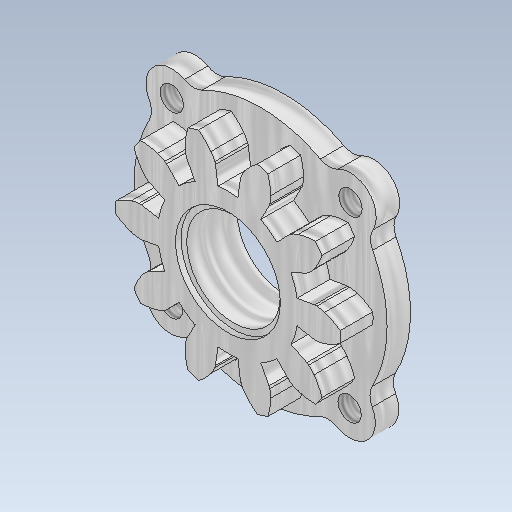
# Autodesk Inventor part: ｍ2歯数10ギア甲d10
Saved by Autodesk Inventor 2020.2 (Build 242310000, 310)
## iProperties
Created: 2019-11-09
Part Number: ｍ2歯数10ギア甲d10
Material: アルミニウム 7075
Document SubType Name: Modeling
Designer: aoyam
Density: 2.81 g/cm^3
Appearance: サテン - ブラシ仕上げ 重厚
Author: aoyam
Autodesk Inventor part; units mm, degrees
ref_plane "YZ Plane" through (0, 0, 0) normal (1, 0, 0) x (0, 1, 0)
ref_plane "XZ Plane" through (0, 0, 0) normal (0, 1, 0) x (-1, 0, 0)
ref_plane "XY Plane" through (0, 0, 0) normal (0, 0, 1) x (1, 0, 0)
sketch "スケッチ1" plane through (0, 0, 0) normal (0, 0, 1) x (1, 0, 0)
  arc A0 (-6.7711, 4.8044) -> (-6.8414, 4.5719) centre (-5.6655, 4.3429) ccw
  arc A1 (-6.3619, 5.5344) -> (-6.7711, 4.8044) centre (-3.6713, 3.5464) ccw
  arc A2 (-5.0279, 6.8503) -> (-6.3619, 5.5344) centre (-1.5449, 1.9856) ccw
  arc A3 (-9.5045, 4.5719) -> (-9.5748, 4.8044) centre (-10.6804, 4.3429) ccw
  arc A4 (-9.5748, 4.8044) -> (-9.984, 5.5344) centre (-12.6746, 3.5464) ccw
  arc A5 (-9.984, 5.5344) -> (-11.318, 6.8503) centre (-14.801, 1.9856) ccw
  arc A6 (-7.1102, 2.6941) -> (-9.2357, 2.6941) centre (-8.1729, -4.7302) ccw
  arc A7 (-11.318, 6.8503) -> (-12.4354, 6.4873) centre (-8.1729, -4.7302) ccw
  line L0 (-7.1102, 2.6941) -> (-6.8414, 4.5719)
  line L1 (-9.2357, 2.6941) -> (-9.5045, 4.5719)
  line L2 (-22.1729, -4.7302) -> (5.8271, -4.7302)
  line L3 (-8.1729, -18.7302) -> (-8.1729, 9.2698)
  arc A8 (-11.6771, 1.9009) -> (-13.3966, 0.6516) centre (-8.1729, -4.7302) ccw
  line L4 (-11.6771, 1.9009) -> (-12.5634, 3.578)
  line L5 (-13.3966, 0.6516) -> (-14.7178, 2.0127)
  arc A9 (-14.7178, 2.0127) -> (-14.9114, 2.1595) centre (-15.5346, 1.1363) ccw
  arc A10 (-12.4354, 6.4873) -> (-12.7411, 4.6385) centre (-6.7582, 4.5989) ccw
  arc A11 (-14.9114, 2.1595) -> (-15.6715, 2.5095) centre (-16.6797, -0.6803) ccw
  arc A12 (-15.6715, 2.5095) -> (-17.5242, 2.7901) centre (-17.4826, -3.1929) ccw
  arc A13 (-17.5242, 2.7901) -> (-18.2148, 1.8395) centre (-8.1729, -4.7302) ccw
  arc A14 (-12.6431, 3.8075) -> (-12.5634, 3.578) centre (-11.4774, 4.084) ccw
  arc A15 (-12.7411, 4.6385) -> (-12.6431, 3.8075) centre (-9.3959, 4.6117) ccw
  arc A16 (-14.9055, -1.4252) -> (-15.5623, -3.4467) centre (-8.1729, -4.7302) ccw
  line L6 (-14.9055, -1.4252) -> (-16.6083, -0.5893)
  line L7 (-15.5623, -3.4467) -> (-17.4312, -3.122)
  arc A17 (-17.4312, -3.122) -> (-17.6741, -3.1171) centre (-17.5768, -4.3112) ccw
  arc A18 (-18.2148, 1.8395) -> (-17.3755, 0.1642) centre (-12.5119, 3.6488) ccw
  arc A19 (-17.6741, -3.1171) -> (-18.4948, -3.2807) centre (-17.4355, -6.4539) ccw
  arc A20 (-18.4948, -3.2807) -> (-20.1586, -4.1427) centre (-16.6083, -8.9586) ccw
  arc A21 (-20.1586, -4.1427) -> (-20.1586, -5.3177) centre (-8.1729, -4.7302) ccw
  arc A22 (-16.8077, -0.4506) -> (-16.6083, -0.5893) centre (-16.0272, 0.4583) ccw
  arc A23 (-17.3755, 0.1642) -> (-16.8077, -0.4506) centre (-14.6534, 2.1087) ccw
  arc A24 (-15.5623, -6.0137) -> (-14.9055, -8.0351) centre (-8.1729, -4.7302) ccw
  line L8 (-15.5623, -6.0137) -> (-17.4312, -6.3384)
  line L9 (-14.9055, -8.0351) -> (-16.6083, -8.871)
  arc A25 (-16.6083, -8.871) -> (-16.8077, -9.0098) centre (-16.0272, -9.9187) ccw
  arc A26 (-20.1586, -5.3177) -> (-18.4948, -6.1797) centre (-16.6083, -0.5018) ccw
  arc A27 (-16.8077, -9.0098) -> (-17.3755, -9.6246) centre (-14.6534, -11.5691) ccw
  arc A28 (-17.3755, -9.6246) -> (-18.2148, -11.2999) centre (-12.5119, -13.1092) ccw
  arc A29 (-18.2148, -11.2999) -> (-17.5242, -12.2504) centre (-8.1729, -4.7302) ccw
  arc A30 (-17.6741, -6.3433) -> (-17.4312, -6.3384) centre (-17.5768, -5.1492) ccw
  arc A31 (-18.4948, -6.1797) -> (-17.6741, -6.3433) centre (-17.4355, -3.0065) ccw
  arc A32 (-13.3966, -10.1119) -> (-11.6771, -11.3612) centre (-8.1729, -4.7302) ccw
  line L10 (-13.3966, -10.1119) -> (-14.7178, -11.4731)
  line L11 (-11.6771, -11.3612) -> (-12.5634, -13.0384)
  arc A33 (-12.5634, -13.0384) -> (-12.6431, -13.2679) centre (-11.4774, -13.5443) ccw
  arc A34 (-17.5242, -12.2504) -> (-15.6715, -11.9699) centre (-17.4826, -6.2675) ccw
  arc A35 (-12.6431, -13.2679) -> (-12.7411, -14.0989) centre (-9.3959, -14.0721) ccw
  arc A36 (-12.7411, -14.0989) -> (-12.4354, -15.9476) centre (-6.7582, -14.0593) ccw
  arc A37 (-12.4354, -15.9476) -> (-11.318, -16.3107) centre (-8.1729, -4.7302) ccw
  arc A38 (-14.9114, -11.6198) -> (-14.7178, -11.4731) centre (-15.5346, -10.5967) ccw
  arc A39 (-15.6715, -11.9699) -> (-14.9114, -11.6198) centre (-16.6797, -8.7801) ccw
  arc A40 (-9.2357, -12.1545) -> (-7.1102, -12.1545) centre (-8.1729, -4.7302) ccw
  line L12 (-9.2357, -12.1545) -> (-9.5045, -14.0323)
  line L13 (-7.1102, -12.1545) -> (-6.8414, -14.0323)
  arc A41 (-6.8414, -14.0323) -> (-6.7711, -14.2648) centre (-5.6655, -13.8033) ccw
  arc A42 (-11.318, -16.3107) -> (-9.984, -14.9948) centre (-14.801, -11.446) ccw
  arc A43 (-6.7711, -14.2648) -> (-6.3619, -14.9948) centre (-3.6713, -13.0068) ccw
  arc A44 (-6.3619, -14.9948) -> (-5.0279, -16.3107) centre (-1.5449, -11.446) ccw
  arc A45 (-5.0279, -16.3107) -> (-3.9105, -15.9476) centre (-8.1729, -4.7302) ccw
  arc A46 (-9.5748, -14.2648) -> (-9.5045, -14.0323) centre (-10.6804, -13.8033) ccw
  arc A47 (-9.984, -14.9948) -> (-9.5748, -14.2648) centre (-12.6746, -13.0068) ccw
  arc A48 (-4.6688, -11.3612) -> (-2.9493, -10.1119) centre (-8.1729, -4.7302) ccw
  line L14 (-4.6688, -11.3612) -> (-3.7825, -13.0384)
  line L15 (-2.9493, -10.1119) -> (-1.6281, -11.4731)
  arc A49 (-1.6281, -11.4731) -> (-1.4345, -11.6198) centre (-0.8113, -10.5967) ccw
  arc A50 (-3.9105, -15.9476) -> (-3.6048, -14.0989) centre (-9.5877, -14.0593) ccw
  arc A51 (-1.4345, -11.6198) -> (-0.6744, -11.9699) centre (0.3338, -8.7801) ccw
  arc A52 (-0.6744, -11.9699) -> (1.1783, -12.2504) centre (1.1367, -6.2675) ccw
  arc A53 (1.1783, -12.2504) -> (1.8689, -11.2999) centre (-8.1729, -4.7302) ccw
  arc A54 (-3.7028, -13.2679) -> (-3.7825, -13.0384) centre (-4.8685, -13.5443) ccw
  arc A55 (-3.6048, -14.0989) -> (-3.7028, -13.2679) centre (-6.95, -14.0721) ccw
  arc A56 (-1.4404, -8.0351) -> (-0.7836, -6.0137) centre (-8.1729, -4.7302) ccw
  line L16 (-1.4404, -8.0351) -> (0.2624, -8.871)
  line L17 (-0.7836, -6.0137) -> (1.0853, -6.3384)
  arc A57 (1.0853, -6.3384) -> (1.3282, -6.3433) centre (1.2309, -5.1492) ccw
  arc A58 (1.8689, -11.2999) -> (1.0296, -9.6246) centre (-3.834, -13.1092) ccw
  arc A59 (1.3282, -6.3433) -> (2.1489, -6.1797) centre (1.0897, -3.0065) ccw
  arc A60 (2.1489, -6.1797) -> (3.8127, -5.3177) centre (0.2624, -0.5018) ccw
  arc A61 (3.8127, -5.3177) -> (3.8127, -4.1427) centre (-8.1729, -4.7302) ccw
  arc A62 (0.4618, -9.0098) -> (0.2624, -8.871) centre (-0.3187, -9.9187) ccw
  arc A63 (1.0296, -9.6246) -> (0.4618, -9.0098) centre (-1.6925, -11.5691) ccw
  arc A64 (-0.7836, -3.4467) -> (-1.4404, -1.4252) centre (-8.1729, -4.7302) ccw
  line L18 (-0.7836, -3.4467) -> (1.0853, -3.122)
  line L19 (-1.4404, -1.4252) -> (0.2624, -0.5893)
  arc A65 (0.2624, -0.5893) -> (0.4618, -0.4506) centre (-0.3187, 0.4583) ccw
  arc A66 (3.8127, -4.1427) -> (2.1489, -3.2807) centre (0.2624, -8.9586) ccw
  arc A67 (0.4618, -0.4506) -> (1.0296, 0.1642) centre (-1.6925, 2.1087) ccw
  arc A68 (1.0296, 0.1642) -> (1.8689, 1.8395) centre (-3.834, 3.6488) ccw
  arc A69 (1.8689, 1.8395) -> (1.1783, 2.7901) centre (-8.1729, -4.7302) ccw
  arc A70 (1.3282, -3.1171) -> (1.0853, -3.122) centre (1.2309, -4.3112) ccw
  arc A71 (2.1489, -3.2807) -> (1.3282, -3.1171) centre (1.0897, -6.4539) ccw
  arc A72 (-2.9493, 0.6516) -> (-4.6688, 1.9009) centre (-8.1729, -4.7302) ccw
  line L20 (-2.9493, 0.6516) -> (-1.6281, 2.0127)
  line L21 (-4.6688, 1.9009) -> (-3.7825, 3.578)
  arc A73 (-3.7825, 3.578) -> (-3.7028, 3.8075) centre (-4.8685, 4.084) ccw
  arc A74 (1.1783, 2.7901) -> (-0.6744, 2.5095) centre (1.1367, -3.1929) ccw
  arc A75 (-3.7028, 3.8075) -> (-3.6048, 4.6385) centre (-6.95, 4.6117) ccw
  arc A76 (-3.6048, 4.6385) -> (-3.9105, 6.4873) centre (-9.5877, 4.5989) ccw
  arc A77 (-3.9105, 6.4873) -> (-5.0279, 6.8503) centre (-8.1729, -4.7302) ccw
  arc A78 (-1.4345, 2.1595) -> (-1.6281, 2.0127) centre (-0.8113, 1.1363) ccw
  arc A79 (-0.6744, 2.5095) -> (-1.4345, 2.1595) centre (0.3338, -0.6803) ccw
  circle A80 centre (-8.1729, -4.7302) radius 2.5
  circle A81 centre (-8.1729, -4.7302) radius 5
  line L22 (-8.1729, -4.7302) -> (-17.6741, 4.8603) construction
  circle A82 centre (-17.6741, 4.8603) radius 1.25
  arc A83 (-16.7463, 5.698) -> (-18.5204, 3.9404) centre (-8.1729, -4.7302) ccw
  arc A84 (-20.0773, 1.6367) -> (-14.4281, 7.2332) centre (-8.1729, -4.7302) ccw
  arc A85 (-16.3313, 7.2602) -> (-20.0865, 3.5401) centre (-17.6741, 4.8603) ccw
  arc A86 (-16.3313, 7.2602) -> (-14.4281, 7.2332) centre (-15.3548, 9.0056) ccw
  arc A87 (-20.0773, 1.6367) -> (-20.0865, 3.5401) centre (-21.8409, 2.5799) ccw
  arc A88 (-20.1633, -12.8886) -> (-20.1364, -10.9853) centre (-21.9087, -11.912) ccw
  arc A89 (-20.1633, -12.8886) -> (-16.4432, -16.6437) centre (-17.7635, -14.2313) ccw
  circle A90 centre (-17.7635, -14.2313) radius 1.25
  arc A91 (-14.5398, -16.6345) -> (-16.4432, -16.6437) centre (-15.483, -18.3981) ccw
  arc A92 (-0.0146, -16.7206) -> (-1.9178, -16.6936) centre (-0.9911, -18.466) ccw
  arc A93 (-0.0146, -16.7206) -> (3.7406, -13.0004) centre (1.3282, -14.3207) ccw
  circle A94 centre (1.3282, -14.3207) radius 1.25
  arc A95 (3.7314, -11.097) -> (3.7406, -13.0004) centre (5.495, -12.0403) ccw
  arc A96 (3.8175, 3.4282) -> (3.7905, 1.5249) centre (5.5628, 2.4516) ccw
  arc A97 (3.8175, 3.4282) -> (0.0973, 7.1833) centre (1.4176, 4.771) ccw
  circle A98 centre (1.4176, 4.771) radius 1.25
  arc A99 (-1.8061, 7.1742) -> (0.0973, 7.1833) centre (-0.8629, 8.9378) ccw
  circle A100 centre (-8.1729, -4.7302) radius 5.6
  point P0 (0, 0)
  point P1 (-16.4019, 6.5961)
  point P2 (-21.4877, -0.4039)
  point P3 (-21.4877, -9.0564)
  point P4 (-16.4019, -16.0564)
  point P5 (-8.1729, -18.7302)
  point P6 (0.056, -16.0564)
  point P7 (5.1418, -9.0564)
  point P8 (5.1418, -0.4039)
  point P9 (0.056, 6.5961)
  point P10 (-18.4948, -3.2807)
  point P11 (-20.1586, -4.1427)
  point P12 (-20.1586, -5.3177)
  point P13 (-18.4948, -6.1797)
  point P14 (-17.6741, -6.3433)
  point P15 (-17.4312, -6.3384)
  point P16 (-15.5623, -6.0137)
  point P17 (-14.9055, -8.0351)
  point P18 (-16.8077, -9.0098)
  point P19 (-17.3755, -9.6246)
  point P20 (-18.2148, -11.2999)
  point P21 (-17.5242, -12.2504)
  point P22 (-15.6715, -11.9699)
  point P23 (-14.9114, -11.6198)
  point P24 (-13.3966, -10.1119)
  point P25 (-11.6771, -11.3612)
  point P26 (-12.5634, -13.0384)
  point P27 (-12.6431, -13.2679)
  point P28 (-12.7411, -14.0989)
  point P29 (-12.4354, -15.9476)
  point P30 (-11.318, -16.3107)
  point P31 (-9.984, -14.9948)
  point P32 (-9.5748, -14.2648)
  point P33 (-9.5045, -14.0323)
  point P34 (-9.2357, -12.1545)
  point P35 (-7.1102, -12.1545)
  point P36 (-6.7711, -14.2648)
  point P37 (-6.3619, -14.9948)
  point P38 (-5.0279, -16.3107)
  point P39 (-3.9105, -15.9476)
  point P40 (-3.6048, -14.0989)
  point P41 (-3.7028, -13.2679)
  point P42 (-3.7825, -13.0384)
  point P43 (-4.6688, -11.3612)
  point P44 (-2.9493, -10.1119)
  point P45 (-1.4345, -11.6198)
  point P46 (-0.6744, -11.9699)
  point P47 (1.1783, -12.2504)
  point P48 (1.8689, -11.2999)
  point P49 (1.0296, -9.6246)
  point P50 (0.4618, -9.0098)
  point P51 (0.2624, -8.871)
  point P52 (-1.4404, -8.0351)
  point P53 (-0.7836, -6.0137)
  point P54 (1.0853, -6.3384)
  point P55 (1.3282, -6.3433)
  point P56 (2.1489, -6.1797)
  point P57 (3.8127, -5.3177)
  point P58 (3.8127, -4.1427)
  point P59 (2.1489, -3.2807)
  point P60 (1.3282, -3.1171)
  point P61 (1.0853, -3.122)
  point P62 (-0.7836, -3.4467)
  point P63 (0.4618, -0.4506)
  point P64 (1.0296, 0.1642)
  point P65 (1.8689, 1.8395)
  point P66 (1.1783, 2.7901)
  point P67 (-0.6744, 2.5095)
  point P68 (-1.4345, 2.1595)
  point P69 (-1.6281, 2.0127)
  point P70 (-2.9493, 0.6516)
  point P71 (-4.6688, 1.9009)
  point P72 (-3.7825, 3.578)
  point P73 (-3.7028, 3.8075)
  point P74 (-3.6048, 4.6385)
  point P75 (-3.9105, 6.4873)
  point P76 (-5.0279, 6.8503)
  point P77 (-6.3619, 5.5344)
  point P78 (-6.7711, 4.8044)
  point P79 (-6.8414, 4.5719)
  point P80 (-7.1102, 2.6941)
  point P81 (-9.2357, 2.6941)
  point P82 (-9.5045, 4.5719)
  point P83 (-9.5748, 4.8044)
  point P84 (-9.984, 5.5344)
  point P85 (-11.318, 6.8503)
  point P86 (-12.4354, 6.4873)
  point P87 (-12.7411, 4.6385)
  point P88 (-12.6431, 3.8075)
  point P89 (-14.9114, 2.1595)
  point P90 (-15.6715, 2.5095)
  point P91 (-17.5242, 2.7901)
  point P92 (-18.2148, 1.8395)
  point P93 (-17.3755, 0.1642)
  point P94 (-16.8077, -0.4506)
  point P95 (-17.6741, -3.1171)
  point P96 (-18.6011, -13.3036)
  point P97 (-16.8436, -15.0777)
  point P98 (0.4004, -15.1584)
  point P99 (2.1745, -13.4008)
  point P100 (2.2552, 3.8432)
  point P101 (0.4977, 5.6173)
  point P102 (-1.9178, -16.6936)
  point P103 (3.7905, 1.5249)
  point P104 (-1.8061, 7.1742)
  point P105 (-20.1364, -10.9853)
  dimension "d2" = 360
  dimension "d6" = 5
  dimension "d8" = 10
  dimension "d9" = 13.5
  dimension "d10" = 2.5
  dimension "d13" = 2
  dimension "d16" = 360
  dimension "d20" = 0.6
  constraints: 196 point on circle, 101 centre point, 46 end point, 5 coincident, 4 tangent, 1 equal radius, 1 midpoint, 442 other
  measures "d6" diameter of A80
  measures "d8" diameter of A81
  measures "d9" distance of L22.start L22.end
  measures "d10" diameter of A82
  measures "d13" radius of A86
  measures "d20" radial gap between concentric circles of A81 A100
extrude "押し出し1" add sketch "スケッチ1" along normal blind 3.5 contours A1 A2 A77 A76 A75 A73 L21 A72 L20 A78 A79 A74 A69 A68 A67 A65 L19 A64 L18 A70 A71 A66 A61 L2 A100 L3 A6 L0 A0 | L3 A100 L2 A21 A20 A19 A17 L7 A16 L6 A22 A23 A18 A13 A12 A11 A9 L5 A8 L4 A14 A15 A10 A7 A5 A4 A3 L1 A6 | A100 L2 A81 L3 | L3 A81 L2 A100 | A100 L3 A81 L2 | L2 A61 A60 A59 A57 L17 A56 L16 A62 A63 A58 A53 A52 A51 A49 L15 A48 L14 A54 A55 A50 A45 A44 A43 A41 L13 A40 L3 A100 | A100 L3 A40 L12 A46 A47 A42 A37 A36 A35 A33 L11 A32 L10 A38 A39 A34 A29 A28 A27 A25 L9 A24 L8 A30 A31 A26 A21 L2 | L2 A81 L3 A100
extrude "押し出し2" add sketch "スケッチ1" against normal blind 2.5 contours A1 A2 A77 A76 A75 A73 L21 A72 L20 A78 A79 A74 A69 A68 A67 A65 L19 A64 L18 A70 A71 A66 A61 L2 A100 L3 A6 L0 A0 | A0 L0 A6 L3 A84 A98 L2 A61 A66 A71 A70 L18 A64 L19 A65 A67 A68 A69 A74 A79 A78 L20 A72 L21 A73 A75 A76 A77 A2 A1 | L3 A100 L2 A21 A20 A19 A17 L7 A16 L6 A22 A23 A18 A13 A12 A11 A9 L5 A8 L4 A14 A15 A10 A7 A5 A4 A3 L1 A6 | A6 L1 A3 A4 A5 A7 A10 A15 A14 L4 A8 L5 A9 A11 A12 A13 A18 A23 A22 L6 A16 L7 A17 A19 A20 A21 L2 A84 A87 A85 A86 L3 | A100 L2 A81 L3 | L3 A81 L2 A100 | A100 L3 A81 L2 | L2 A61 A60 A59 A57 L17 A56 L16 A62 A63 A58 A53 A52 A51 A49 L15 A48 L14 A54 A55 A50 A45 A44 A43 A41 L13 A40 L3 A100 | A100 L3 A40 L12 A46 A47 A42 A37 A36 A35 A33 L11 A32 L10 A38 A39 A34 A29 A28 A27 A25 L9 A24 L8 A30 A31 A26 A21 L2 | L2 A81 L3 A100 | A99 A97 A96 A84 A98 | L2 A84 A94 L3 A40 L13 A41 A43 A44 A45 A50 A55 A54 L14 A48 L15 A49 A51 A52 A53 A58 A63 A62 L16 A56 L17 A57 A59 A60 A61 | A21 A26 A31 A30 L8 A24 L9 A25 A27 A28 A29 A34 A39 A38 L10 A32 L11 A33 A35 A36 A37 A42 A47 A46 L12 A40 L3 A84 A90 L2 | A95 A93 A92 A84 A94 | A84 A90 A91 A89 A88
sketch "スケッチ3" plane through (0, 0, -2.5) normal (0, 0, -1) x (-1, 0, 0)
  circle A0 centre (8.1729, -4.7302) radius 5 projected
  circle A1 centre (8.1729, -4.7302) radius 5.6
  point P0 (0, 0)
  dimension "d21" = 0.6
  constraints: 1 centre point
  measures "d21" radial gap between concentric circles of A0 A1
sketch "スケッチ4" plane through (0, 0, 3.5) normal (0, 0, 1) x (1, 0, 0)
  circle A0 centre (-8.1729, -4.7302) radius 5 projected
  circle A1 centre (-8.1729, -4.7302) radius 5.6
  point P0 (0, 0)
  dimension "d22" = 0.6
  constraints: 1 centre point
  measures "d22" radial gap between concentric circles of A0 A1
extrude "押し出し3" cut sketch "スケッチ4" against normal blind 0.6
sketch "スケッチ5" plane through (0, 0, 3.5) normal (0, 0, 1) x (1, 0, 0)
  circle A0 centre (-17.7635, -14.2313) radius 1.25 projected
  circle A1 centre (-17.6741, 4.8603) radius 1.25 projected
  circle A2 centre (1.3282, -14.3207) radius 1.25 projected
  circle A3 centre (1.4176, 4.771) radius 1.25 projected
  arc A4 (3.7314, -11.097) -> (3.7905, 1.5249) centre (-8.1729, -4.7302) ccw projected
  arc A5 (3.8175, 3.4282) -> (3.7905, 1.5249) centre (5.5628, 2.4516) ccw projected
  arc A6 (3.8175, 3.4282) -> (0.0973, 7.1833) centre (1.4176, 4.771) ccw projected
  arc A7 (-1.8061, 7.1742) -> (0.0973, 7.1833) centre (-0.8629, 8.9378) ccw projected
  arc A8 (-1.8061, 7.1742) -> (-14.4281, 7.2332) centre (-8.1729, -4.7302) ccw projected
  arc A9 (-16.3313, 7.2602) -> (-14.4281, 7.2332) centre (-15.3548, 9.0056) ccw projected
  arc A10 (-16.3313, 7.2602) -> (-20.0865, 3.5401) centre (-17.6741, 4.8603) ccw projected
  arc A11 (-20.0773, 1.6367) -> (-20.0865, 3.5401) centre (-21.8409, 2.5799) ccw projected
  arc A12 (-20.0773, 1.6367) -> (-20.1364, -10.9853) centre (-8.1729, -4.7302) ccw projected
  arc A13 (-20.1633, -12.8886) -> (-20.1364, -10.9853) centre (-21.9087, -11.912) ccw projected
  arc A14 (-20.1633, -12.8886) -> (-16.4432, -16.6437) centre (-17.7635, -14.2313) ccw projected
  arc A15 (-14.5398, -16.6345) -> (-16.4432, -16.6437) centre (-15.483, -18.3981) ccw projected
  arc A16 (-14.5398, -16.6345) -> (-1.9178, -16.6936) centre (-8.1729, -4.7302) ccw projected
  arc A17 (-0.0146, -16.7206) -> (-1.9178, -16.6936) centre (-0.9911, -18.466) ccw projected
  arc A18 (-0.0146, -16.7206) -> (3.7406, -13.0004) centre (1.3282, -14.3207) ccw projected
  arc A19 (3.7314, -11.097) -> (3.7406, -13.0004) centre (5.495, -12.0403) ccw projected
  line L0 (-11.6771, -11.3612) -> (-12.5634, -13.0384) projected
  arc A20 (-13.3966, -10.1119) -> (-11.6771, -11.3612) centre (-8.1729, -4.7302) ccw projected
  line L1 (-14.7178, -11.4731) -> (-13.3966, -10.1119) projected
  arc A21 (-14.9114, -11.6198) -> (-14.7178, -11.4731) centre (-15.5346, -10.5967) ccw projected
  arc A22 (-15.6715, -11.9699) -> (-14.9114, -11.6198) centre (-16.6797, -8.7801) ccw projected
  arc A23 (-17.5242, -12.2504) -> (-15.6715, -11.9699) centre (-17.4826, -6.2675) ccw projected
  arc A24 (-18.2148, -11.2999) -> (-17.5242, -12.2504) centre (-8.1729, -4.7302) ccw projected
  arc A25 (-17.3755, -9.6246) -> (-18.2148, -11.2999) centre (-12.5119, -13.1092) ccw projected
  arc A26 (-16.8077, -9.0098) -> (-17.3755, -9.6246) centre (-14.6534, -11.5691) ccw projected
  arc A27 (-16.6083, -8.871) -> (-16.8077, -9.0098) centre (-16.0272, -9.9187) ccw projected
  line L2 (-14.9055, -8.0351) -> (-16.6083, -8.871) projected
  arc A28 (-15.5623, -6.0137) -> (-14.9055, -8.0351) centre (-8.1729, -4.7302) ccw projected
  line L3 (-17.4312, -6.3384) -> (-15.5623, -6.0137) projected
  arc A29 (-17.6741, -6.3433) -> (-17.4312, -6.3384) centre (-17.5768, -5.1492) ccw projected
  arc A30 (-18.4948, -6.1797) -> (-17.6741, -6.3433) centre (-17.4355, -3.0065) ccw projected
  arc A31 (-20.1586, -5.3177) -> (-18.4948, -6.1797) centre (-16.6083, -0.5018) ccw projected
  arc A32 (-20.1586, -4.1427) -> (-20.1586, -5.3177) centre (-8.1729, -4.7302) ccw projected
  arc A33 (-18.4948, -3.2807) -> (-20.1586, -4.1427) centre (-16.6083, -8.9586) ccw projected
  arc A34 (-17.6741, -3.1171) -> (-18.4948, -3.2807) centre (-17.4355, -6.4539) ccw projected
  arc A35 (-17.4312, -3.122) -> (-17.6741, -3.1171) centre (-17.5768, -4.3112) ccw projected
  line L4 (-15.5623, -3.4467) -> (-17.4312, -3.122) projected
  arc A36 (-14.9055, -1.4252) -> (-15.5623, -3.4467) centre (-8.1729, -4.7302) ccw projected
  line L5 (-16.6083, -0.5893) -> (-14.9055, -1.4252) projected
  arc A37 (-16.8077, -0.4506) -> (-16.6083, -0.5893) centre (-16.0272, 0.4583) ccw projected
  arc A38 (-17.3755, 0.1642) -> (-16.8077, -0.4506) centre (-14.6534, 2.1087) ccw projected
  arc A39 (-18.2148, 1.8395) -> (-17.3755, 0.1642) centre (-12.5119, 3.6488) ccw projected
  arc A40 (-17.5242, 2.7901) -> (-18.2148, 1.8395) centre (-8.1729, -4.7302) ccw projected
  arc A41 (-15.6715, 2.5095) -> (-17.5242, 2.7901) centre (-17.4826, -3.1929) ccw projected
  arc A42 (-14.9114, 2.1595) -> (-15.6715, 2.5095) centre (-16.6797, -0.6803) ccw projected
  arc A43 (-14.7178, 2.0127) -> (-14.9114, 2.1595) centre (-15.5346, 1.1363) ccw projected
  line L6 (-13.3966, 0.6516) -> (-14.7178, 2.0127) projected
  arc A44 (-11.6771, 1.9009) -> (-13.3966, 0.6516) centre (-8.1729, -4.7302) ccw projected
  line L7 (-12.5634, 3.578) -> (-11.6771, 1.9009) projected
  arc A45 (-12.6431, 3.8075) -> (-12.5634, 3.578) centre (-11.4774, 4.084) ccw projected
  arc A46 (-12.7411, 4.6385) -> (-12.6431, 3.8075) centre (-9.3959, 4.6117) ccw projected
  arc A47 (-12.4354, 6.4873) -> (-12.7411, 4.6385) centre (-6.7582, 4.5989) ccw projected
  arc A48 (-11.318, 6.8503) -> (-12.4354, 6.4873) centre (-8.1729, -4.7302) ccw projected
  arc A49 (-9.984, 5.5344) -> (-11.318, 6.8503) centre (-14.801, 1.9856) ccw projected
  arc A50 (-9.5748, 4.8044) -> (-9.984, 5.5344) centre (-12.6746, 3.5464) ccw projected
  arc A51 (-9.5045, 4.5719) -> (-9.5748, 4.8044) centre (-10.6804, 4.3429) ccw projected
  line L8 (-9.2357, 2.6941) -> (-9.5045, 4.5719) projected
  arc A52 (-7.1102, 2.6941) -> (-9.2357, 2.6941) centre (-8.1729, -4.7302) ccw projected
  line L9 (-6.8414, 4.5719) -> (-7.1102, 2.6941) projected
  arc A53 (-6.7711, 4.8044) -> (-6.8414, 4.5719) centre (-5.6655, 4.3429) ccw projected
  arc A54 (-6.3619, 5.5344) -> (-6.7711, 4.8044) centre (-3.6713, 3.5464) ccw projected
  arc A55 (-5.0279, 6.8503) -> (-6.3619, 5.5344) centre (-1.5449, 1.9856) ccw projected
  arc A56 (-3.9105, 6.4873) -> (-5.0279, 6.8503) centre (-8.1729, -4.7302) ccw projected
  arc A57 (-3.6048, 4.6385) -> (-3.9105, 6.4873) centre (-9.5877, 4.5989) ccw projected
  arc A58 (-3.7028, 3.8075) -> (-3.6048, 4.6385) centre (-6.95, 4.6117) ccw projected
  arc A59 (-3.7825, 3.578) -> (-3.7028, 3.8075) centre (-4.8685, 4.084) ccw projected
  line L10 (-4.6688, 1.9009) -> (-3.7825, 3.578) projected
  arc A60 (-2.9493, 0.6516) -> (-4.6688, 1.9009) centre (-8.1729, -4.7302) ccw projected
  line L11 (-1.6281, 2.0127) -> (-2.9493, 0.6516) projected
  arc A61 (-1.4345, 2.1595) -> (-1.6281, 2.0127) centre (-0.8113, 1.1363) ccw projected
  arc A62 (-0.6744, 2.5095) -> (-1.4345, 2.1595) centre (0.3338, -0.6803) ccw projected
  arc A63 (1.1783, 2.7901) -> (-0.6744, 2.5095) centre (1.1367, -3.1929) ccw projected
  arc A64 (1.8689, 1.8395) -> (1.1783, 2.7901) centre (-8.1729, -4.7302) ccw projected
  arc A65 (1.0296, 0.1642) -> (1.8689, 1.8395) centre (-3.834, 3.6488) ccw projected
  arc A66 (0.4618, -0.4506) -> (1.0296, 0.1642) centre (-1.6925, 2.1087) ccw projected
  arc A67 (0.2624, -0.5893) -> (0.4618, -0.4506) centre (-0.3187, 0.4583) ccw projected
  line L12 (-1.4404, -1.4252) -> (0.2624, -0.5893) projected
  arc A68 (-0.7836, -3.4467) -> (-1.4404, -1.4252) centre (-8.1729, -4.7302) ccw projected
  line L13 (1.0853, -3.122) -> (-0.7836, -3.4467) projected
  arc A69 (1.3282, -3.1171) -> (1.0853, -3.122) centre (1.2309, -4.3112) ccw projected
  arc A70 (2.1489, -3.2807) -> (1.3282, -3.1171) centre (1.0897, -6.4539) ccw projected
  arc A71 (3.8127, -4.1427) -> (2.1489, -3.2807) centre (0.2624, -8.9586) ccw projected
  arc A72 (3.8127, -5.3177) -> (3.8127, -4.1427) centre (-8.1729, -4.7302) ccw projected
  arc A73 (2.1489, -6.1797) -> (3.8127, -5.3177) centre (0.2624, -0.5018) ccw projected
  arc A74 (1.3282, -6.3433) -> (2.1489, -6.1797) centre (1.0897, -3.0065) ccw projected
  arc A75 (1.0853, -6.3384) -> (1.3282, -6.3433) centre (1.2309, -5.1492) ccw projected
  line L14 (-0.7836, -6.0137) -> (1.0853, -6.3384) projected
  arc A76 (-1.4404, -8.0351) -> (-0.7836, -6.0137) centre (-8.1729, -4.7302) ccw projected
  line L15 (0.2624, -8.871) -> (-1.4404, -8.0351) projected
  arc A77 (0.4618, -9.0098) -> (0.2624, -8.871) centre (-0.3187, -9.9187) ccw projected
  arc A78 (1.0296, -9.6246) -> (0.4618, -9.0098) centre (-1.6925, -11.5691) ccw projected
  arc A79 (1.8689, -11.2999) -> (1.0296, -9.6246) centre (-3.834, -13.1092) ccw projected
  arc A80 (1.1783, -12.2504) -> (1.8689, -11.2999) centre (-8.1729, -4.7302) ccw projected
  arc A81 (-0.6744, -11.9699) -> (1.1783, -12.2504) centre (1.1367, -6.2675) ccw projected
  arc A82 (-1.4345, -11.6198) -> (-0.6744, -11.9699) centre (0.3338, -8.7801) ccw projected
  arc A83 (-1.6281, -11.4731) -> (-1.4345, -11.6198) centre (-0.8113, -10.5967) ccw projected
  line L16 (-2.9493, -10.1119) -> (-1.6281, -11.4731) projected
  arc A84 (-4.6688, -11.3612) -> (-2.9493, -10.1119) centre (-8.1729, -4.7302) ccw projected
  line L17 (-3.7825, -13.0384) -> (-4.6688, -11.3612) projected
  arc A85 (-3.7028, -13.2679) -> (-3.7825, -13.0384) centre (-4.8685, -13.5443) ccw projected
  arc A86 (-3.6048, -14.0989) -> (-3.7028, -13.2679) centre (-6.95, -14.0721) ccw projected
  arc A87 (-3.9105, -15.9476) -> (-3.6048, -14.0989) centre (-9.5877, -14.0593) ccw projected
  arc A88 (-5.0279, -16.3107) -> (-3.9105, -15.9476) centre (-8.1729, -4.7302) ccw projected
  arc A89 (-6.3619, -14.9948) -> (-5.0279, -16.3107) centre (-1.5449, -11.446) ccw projected
  arc A90 (-6.7711, -14.2648) -> (-6.3619, -14.9948) centre (-3.6713, -13.0068) ccw projected
  arc A91 (-6.8414, -14.0323) -> (-6.7711, -14.2648) centre (-5.6655, -13.8033) ccw projected
  line L18 (-7.1102, -12.1545) -> (-6.8414, -14.0323) projected
  arc A92 (-9.2357, -12.1545) -> (-7.1102, -12.1545) centre (-8.1729, -4.7302) ccw projected
  line L19 (-9.5045, -14.0323) -> (-9.2357, -12.1545) projected
  arc A93 (-9.5748, -14.2648) -> (-9.5045, -14.0323) centre (-10.6804, -13.8033) ccw projected
  arc A94 (-9.984, -14.9948) -> (-9.5748, -14.2648) centre (-12.6746, -13.0068) ccw projected
  arc A95 (-11.318, -16.3107) -> (-9.984, -14.9948) centre (-14.801, -11.446) ccw projected
  arc A96 (-12.4354, -15.9476) -> (-11.318, -16.3107) centre (-8.1729, -4.7302) ccw projected
  arc A97 (-12.7411, -14.0989) -> (-12.4354, -15.9476) centre (-6.7582, -14.0593) ccw projected
  arc A98 (-12.6431, -13.2679) -> (-12.7411, -14.0989) centre (-9.3959, -14.0721) ccw projected
  arc A99 (-12.5634, -13.0384) -> (-12.6431, -13.2679) centre (-11.4774, -13.5443) ccw projected
  circle A100 centre (-8.1729, -4.7302) radius 5.6 projected
  circle A101 centre (-8.1729, -4.7302) radius 5 projected
  circle A102 centre (-8.1729, -4.7302) radius 12
  circle A103 centre (-8.1729, -4.7302) radius 16.25
  point P0 (0, 0)
  point P1 (1.3282, 3.5242)
  dimension "d28" = 32.5
  constraints: 2 coincident, 1 centre point, 5 other
  measures "d28" diameter of A103
thread "ねじ1" size "M3x0.5" class "6H" standard "ANSI Metric M Profile" full length
thread "ねじ2" size "M3x0.5" class "6H" standard "ANSI Metric M Profile" full length
thread "ねじ3" size "M3x0.5" class "6H" standard "ANSI Metric M Profile" full length
thread "ねじ4" size "M3x0.5" class "6H" standard "ANSI Metric M Profile" full length
